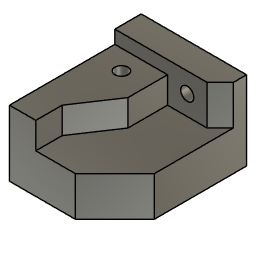
Robocon Task 1C 1 (Autodesk Fusion 360 design; units mm, degrees)
Autodesk Fusion 360 part; units mm, degrees
sketch "Sketch1" plane through (0, 0, 0) normal (0, 0, 1) x (1, 0, 0)
  line L0 (0, 0) -> (16, 0)
  line L1 (16, 0) -> (16, -14)
  line L2 (0, -20) -> (10, -20)
  line L3 (0, -20) -> (0, 0)
  line L4 (10, -20) -> (16, -14)
  dimension "d1" = 16
  dimension "d2" = 14
  dimension "d3" = 10
  dimension "d4" = 20
  constraint coincident L0.start L3.end
  constraint horizontal L0
  constraint perpendicular L0 L1
  constraint horizontal L2
  constraint perpendicular L0 L3
  measures "d1" distance of L0.start L0.end
  measures "d2" distance of L0.end L1.end
  measures "d3" distance of L2.start L2.end
  measures "d4" distance of L2.start L0.start
extrude "Extrude1" add sketch "Sketch1" along normal blind 6
sketch "Sketch2" plane through (0, 0, 6) normal (0, 0, 1) x (-1, 0, 0)
  line L0 (0, 20) -> (-10, 20)
  line L1 (-10, 20) -> (-16, 14)
  line L2 (-16, 14) -> (-16, 0)
  line L3 (-16, 0) -> (0, 0)
  line L4 (0, 0) -> (0, 20)
  line L5 (0, 0) -> (-14, 0)
  line L6 (-14, 0) -> (-14, 4)
  line L7 (-14, 4) -> (0, 4)
  line L8 (0, 4) -> (0, 0)
  line L9 (-14, 4) -> (-16, 2)
  line L10 (-14, 4) -> (-11.1716, 4) construction
  line L11 (0, 20) -> (-4, 20)
  line L12 (-4, 20) -> (-4, 4)
  line L13 (-4, 4) -> (0, 4)
  line L14 (0, 4) -> (0, 20)
  line L15 (0, 4) -> (-8, 4)
  line L16 (-8, 4) -> (-8, 10)
  line L17 (-8, 10) -> (0, 10)
  line L18 (0, 10) -> (0, 4)
  line L19 (-8, 10) -> (-4, 16)
  dimension "d7" = 14
  dimension "d8" = 4
  dimension "d9" = 135
  dimension "d10" = 4
  dimension "d11" = 8
  dimension "d12" = 6
  dimension "d13" = 4
  constraint horizontal L5
  constraint vertical L6
  constraint horizontal L7
  constraint vertical L8
  constraint coincident L3.end L4.start
  constraint horizontal L10
  constraint coincident L2 L9.end
  constraint horizontal L11
  constraint vertical L12
  constraint horizontal L13
  constraint vertical L14
  constraint coincident L0.start L4.end
  constraint horizontal L15
  constraint vertical L16
  constraint horizontal L17
  constraint vertical L18
  constraint coincident L12 L19.end
  measures "d7" distance of L3.end L5.end
  measures "d8" distance of L3.end L7.end
  measures "d9" angle of L9 L10
  measures "d10" distance of L0.start L11.end
  measures "d11" distance of L7.end L15.end
  measures "d12" distance of L7.end L17.end
  measures "d13" distance of L0 L19.end
extrude "Extrude2" add sketch "Sketch2" along normal blind 4 contours L0 L4 L11 L12 L14 L17 | L4 L7 L12 L13 L14 L15 L17 L18 | L12 L17 L19 | L7 L12 L15 L16 L17
extrude "Extrude3" add sketch "Sketch2" along normal blind 6 contours L3 L4 L5 L6 L7 L8 L13 L15 | L2 L3 L6 L9
sketch "Sketch3" plane through (0, -4, 0) normal (0, -1, 0) x (1, 0, 0)
  line L0 (0, 10) -> (8, 10)
  line L1 (8, 10) -> (8, 6)
  line L2 (8, 6) -> (14, 6)
  line L3 (14, 6) -> (14, 12)
  line L4 (14, 12) -> (0, 12)
  line L5 (0, 12) -> (0, 10)
  circle A0 centre (11, 9) radius 1
  dimension "d18" = 2
  dimension "d19" = 3
  dimension "d20" = 3
  measures "d18" diameter of A0
  measures "d19" distance of L3 A0.centre
  measures "d20" distance of L2 A0.centre
extrude "Extrude4" cut sketch "Sketch3" against normal blind 9 contours A0
sketch "Sketch4" plane through (0, 0, 10) normal (0, 0, 1) x (-1, 0, 0)
  line L0 (0, 4) -> (0, 20)
  line L1 (0, 20) -> (-4, 20)
  line L2 (-4, 20) -> (-4, 16)
  line L3 (-4, 16) -> (-8, 10)
  line L4 (-8, 10) -> (-8, 4)
  line L5 (-8, 4) -> (0, 4)
  circle A0 centre (-4, 7) radius 1
  dimension "d23" = 2
  dimension "d24" = 4
  dimension "d25" = 3
  measures "d23" diameter of A0
  measures "d24" distance of L4 A0.centre
  measures "d25" distance of L5 A0.centre
extrude "Extrude5" cut sketch "Sketch4" against normal blind 9.5 contours A0
